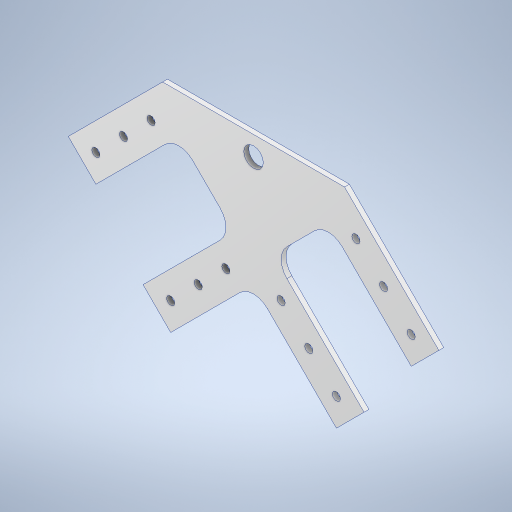
# Autodesk Inventor part: KneePivotPlate
Saved by Autodesk Inventor 2023 (Build 270158000, 158)
## iProperties
Created: 2023-03-03
Part Number: KneePivotPlate
Material: Aluminum 6061
Document SubType Name: Modeling
Designer: megan
Density: 2.7 g/cm^3
Appearance: Aluminum - Flat
Mass: 113.282 g
Surface Area: 301.739 cm^2
Volume: 41.9562 cm^3
Author: megan
Autodesk Inventor part; units mm, degrees
ref_plane "YZ Plane" through (0, 0, 0) normal (1, 0, 0) x (0, 1, 0)
ref_plane "XZ Plane" through (0, 0, 0) normal (0, 1, 0) x (-1, 0, 0)
ref_plane "XY Plane" through (0, 0, 0) normal (0, 0, 1) x (1, 0, 0)
sketch "Sketch8" plane through (0, 0, 0) normal (0, 0, 1) x (1, 0, 0)
  circle A0 centre (0, 0) radius 6.35
  line L0 (0, -153.4083) -> (0, 40.3847) projected
  line L1 (0, 12.7) -> (59.142, 12.7)
  line L2 (59.142, 12.7) -> (120.4631, -48.621)
  line L3 (120.4631, -48.621) -> (102.5026, -66.5815)
  line L4 (102.5026, -66.5815) -> (48.621, -12.7)
  line L5 (0, 0) -> (88.4811, -88.4811) construction
  line L6 (48.621, -12.7) -> (12.7, -48.621)
  line L7 (0, 12.7) -> (-59.142, 12.7)
  line L8 (-59.142, 12.7) -> (-120.4631, -48.621)
  line L9 (-120.4631, -48.621) -> (-102.5026, -66.5815)
  line L10 (-102.5026, -66.5815) -> (-48.621, -12.7)
  line L11 (0, 0) -> (-88.4811, -88.4811) construction
  line L12 (-48.621, -12.7) -> (-12.7, -48.621)
  line L13 (0, -71.842) -> (53.8815, -125.7236)
  line L14 (53.8815, -125.7236) -> (71.842, -107.7631)
  line L15 (71.842, -107.7631) -> (12.7, -48.621)
  line L16 (0, -71.842) -> (-53.8815, -125.7236)
  line L17 (-53.8815, -125.7236) -> (-71.842, -107.7631)
  line L18 (-71.842, -107.7631) -> (-12.7, -48.621)
  dimension "d108" = 12.7
  dimension "d110" = 25.4
  dimension "d111" = 76.2
  dimension "d112" = 12.7
  dimension "d113" = 12.7
  dimension "d114" = 50.8
  dimension "d115" = 135
  dimension "d131" = 76.2
  dimension "d133" = 25.4
  constraints: 36 end point, 9 symmetric about line, 3 parallel, 3 perpendicular, 2 point on line, 1 centre point, 1 coincident, 1 horizontal
  measures "d108" diameter of A0
  measures "d110" distance of L2.end L3.end
  measures "d111" distance of L3.end L4.end
  measures "d112" distance from line of L1 point (0, 0)
  measures "d113" vertical distance of L4.end point (0, 0)
  measures "d114" distance between parallel lines of L5 L2
  measures "d115" angle of L2 L1
  measures "d131" distance of L13.start L13.end
  measures "d133" distance of L13.end L14.end
extrude "Extrusion6" add sketch "Sketch8" along normal mid plane 3.175 contours A0 L0 L1 L2 L3 L4 L6 L15 L14 L13 | A0 L0 L16 L17 L18 L12 L10 L9 L8 L7
sketch "Sketch9" plane through (0, 0, 1.5875) normal (0, 0, 1) x (1, 0, 0)
  line L0 (-59.142, 12.7) -> (-120.4631, -48.621) projected
  line L1 (-102.5026, -66.5815) -> (-48.621, -12.7) projected
  line L2 (-120.4631, -66.5815) -> (0, 53.8815) construction
  line L3 (0, -161.6446) -> (0, 89.8026) construction
  circle A0 centre (-102.5026, -48.621) radius 2.65
  line L4 (-120.4631, -48.621) -> (-102.5026, -66.5815) construction
  circle A1 centre (-84.542, -30.6605) radius 2.65
  circle A2 centre (-66.5815, -12.7) radius 2.65
  line L5 (-93.5249, -93.5249) -> (0, 0) construction
  line L6 (-71.842, -125.7236) -> (0, -53.8815) construction
  line L7 (-12.7, -48.621) -> (-71.842, -107.7631) construction
  circle A3 centre (-53.8815, -107.7631) radius 2.65
  line L8 (-71.842, -107.7631) -> (-53.8815, -125.7236) construction
  circle A4 centre (-35.921, -89.8026) radius 2.65
  circle A5 centre (-17.9605, -71.842) radius 2.65
  dimension "d119" = 45
  dimension "d120" = 12.7
  dimension "d121" = 5.3
  dimension "d124" = 25.4
  dimension "d134" = 5.3
  dimension "d135" = 12.7
  dimension "d138" = 25.4
  constraints: 6 centre point, 6 end point, 3 point on line, 2 parallel, 10 other
  measures "d119" angle of L3 L2
  measures "d120" distance from line of L4 A0.centre
  measures "d121" diameter of A0
  measures "d124" distance of A0.centre A1.centre
  measures "d134" diameter of A3
  measures "d135" distance from line of L8 A3.centre
  measures "d138" distance of A3.centre A4.centre
extrude "Extrusion7" cut sketch "Sketch9" against normal blind 25.4
mirror "Mirror3" about plane through (0, 0, 0) normal (1, 0, 0) of "Extrusion7"
fillet "Fillet4" radius 12.7 5 edges at (-48.621, -12.7, 0) (48.621, -12.7, 0) (0, -71.842, 0) (-12.7, -48.621, 0) (12.7, -48.621, 0)
equation "\"topDiameter\" = 45"
equation "\"bearingDiameter\" = 28.62"
equation "\"plateThickness\" = 6.35"
equation "\"theta12\" = 90deg"
equation "\"gearboxLength\" = 101.6"
equation "\"boltedLength\" = 76.2"
equation "\"topDiameter_1\" = 25"
equation "\"shaftLength_1\" = 76.2"
equation "\"bearingDiameter_1\" = 28.62"
equation "\"plateThickness_1\" = 6.35"
equation "\"theta12_1\" = 100deg"
equation "\"boltDiameter_1\" = 6"
equation "\"gearboxLength_1\" = 101.6"
equation "\"boltedLength_1\" = 76.2"
equation "\"innerBoltSpacing_1\" = 12.7"
equation "\"outerBoltSpacing_1\" = 12.7"
equation "\"shaftLength\" = 76.2"
equation "\"boltDiameter\" = 5.3"
equation "\"outerBoltSpacing\" = 12.7"
equation "\"innerBoltSpacing\" = 12.7"
body "Solid1"
